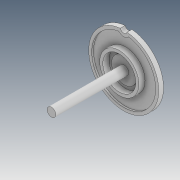
# Autodesk Inventor part: PMSeal
Saved by Autodesk Inventor 2020 (Build 240168000, 168)
## iProperties
Created: 2020-05-07
Part Number: PMSeal
Material: Generic
Document SubType Name: Modeling
Designer: Theo Cominotto
Density: 1 g/cm^3
Appearance: Default
Author: Theo Cominotto
Autodesk Inventor part; units mm, degrees
sketch "Sketch1" plane through (0, 0, 0) normal (0, 0, 1) x (1, 0, 0)
  circle A0 centre (0, 0) radius 11.4
  dimension "d0" = 22.8
  constraints: 1 centre point, 1 coincident
  measures "d0" diameter of A0
extrude "Extrusion1" add sketch "Sketch1" along normal blind 1
ref_plane "Work Plane1" through (0, 0, 1) normal (0, 0, 1) x (1, 0, 0)
sketch "Sketch3" plane through (0, 0, 1) normal (0, 0, 1) x (1, 0, 0)
  circle A0 centre (0, 0) radius 6.375
  circle A1 centre (0, 0) radius 5.375
  dimension "d6" = 12.75
  dimension "d7" = 10.75
  constraints: 2 centre point, 2 coincident
  measures "d6" diameter of A0
  measures "d7" diameter of A1
extrude "Extrusion3" add sketch "Sketch3" along normal blind 2
ref_plane "Work Plane3" through (0, 0, 1) normal (0, 0, 1) x (1, 0, 0)
sketch "Sketch4" plane through (0, 0, 1) normal (0, 0, 1) x (1, 0, 0)
  circle A0 centre (0, 0) radius 1.425
  dimension "d10" = 2.85
  constraints: 1 centre point, 1 coincident
  measures "d10" diameter of A0
extrude "Extrusion4" add sketch "Sketch4" along normal blind 24.1
ref_plane "Work Plane2" through (0, 0, 1) normal (0, 0, 1) x (1, 0, 0)
sketch "Sketch5" plane through (0, 0, 1) normal (0, 0, 1) x (1, 0, 0)
  circle A0 centre (0, 0) radius 4.125
  dimension "d14" = 8.25
  constraints: 1 centre point, 1 coincident
  measures "d14" diameter of A0
extrude "Extrusion5" add sketch "Sketch5" along normal blind 0.4
sketch "Sketch7" plane through (0, 0, 1) normal (0, 0, 1) x (1, 0, 0)
  circle A0 centre (0, 0) radius 11.4
  line L0 (-1.1, 11.3468) -> (1.1, 11.3468) construction
  line L1 (0, 11.3468) -> (0, 10.5468) construction
  arc A1 (-1.1, 11.3468) -> (1.1, 11.3468) centre (0, 11.7031) ccw
  dimension "d17" = 2.2
  dimension "d18" = 0.8
  constraints: 5 point on circle, 4 end point, 2 centre point, 1 horizontal, 1 midpoint, 1 vertical
  measures "d17" distance of L0.start L0.end
  measures "d18" distance of L1.start L1.end
extrude "Extrusion6" cut sketch "Sketch7" against normal up to surface (1 mm away) contours A1 A0 picked at (-0.044, 11.1142)
sketch "Sketch8" plane through (0, 0, 1) normal (0, 0, 1) x (1, 0, 0)
  arc A0 (-1.1, 11.3468) -> (1.1, 11.3468) centre (0, 11.7031) ccw projected
  arc A1 (-1.1, 11.3468) -> (1.1, 11.3468) centre (0, 0) ccw projected
  circle A2 centre (0, 0) radius 6.375 projected
  arc A3 (-1.6146, 10.2739) -> (1.6146, 10.2739) centre (0, 11.7031) ccw
  arc A4 (-1.6146, 10.2739) -> (1.6146, 10.2739) centre (0, 0) ccw
  dimension "d21" = 1
  constraints: 4 point on circle, 2 centre point, 1 other
  measures "d21" radial gap between concentric circles of A1 A4
extrude "Extrusion7" add sketch "Sketch8" along normal blind 0.57 contours A0 A1
body "Solid1"
